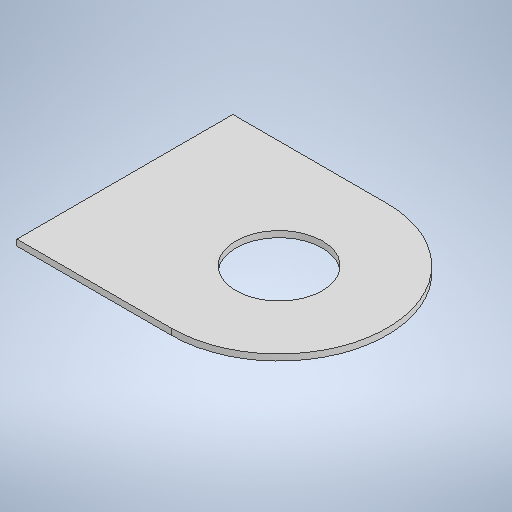
# Autodesk Inventor part: AKVA MSC 0512 transverse ring1 4mm 304 8pcs
Saved by Autodesk Inventor 2025 (Build 290162010, 162A)
## iProperties
Created: 2024-07-11
Part Number: AKVA MSC 0512 transverse ring1 4mm 304 8pcs
Material: Stainless Steel
Document SubType Name: Sheet Metal
Designer: admin
Density: 8 g/cm^3
Sheet Metal Rule: AISI304 2mm Die16
Sheet Metal Width: 85,000 mm
Sheet Metal Length: 70,000 mm
Sheet Metal Area: 5950,000 mm^2
Appearance: Default
Flat Pattern Width: 8.5 cm
Flat Pattern Length: 7 cm
Flat Pattern Area: 59.5 cm^2
Author: admin
Autodesk Inventor part; units mm, degrees
ref_plane "YZ Plane" through (0, 0, 0) normal (1, 0, 0) x (0, 1, 0)
ref_plane "XZ Plane" through (0, 0, 0) normal (0, 1, 0) x (-1, 0, 0)
ref_plane "XY Plane" through (0, 0, 0) normal (0, 0, 1) x (1, 0, 0)
sketch "Sketch1" plane through (0, 0, 0) normal (0, 0, 1) x (1, 0, 0)
  line L0 (0, 35) -> (0, -35)
  line L1 (0, -35) -> (50, -35)
  line L2 (50, 35) -> (0, 35)
  circle A0 centre (50, 0) radius 14
  arc A1 (50, -35) -> (50, 35) centre (50, 0) ccw
  point P0 (0, 0)
  point P1 (0, 0)
  dimension "d11" = 70
  dimension "d12" = 50
  dimension "d14" = 28
  measures "d11" distance of L0.start L0.end
  measures "d12" distance of L0.end L1.end
  measures "d14" diameter of A0
extrude "Plate1" add sketch "Sketch1" along normal blind 2
equation "\"d5\" = Thickness"
equation "\"BendReliefWidth\" = Thickness"
equation "\"BendReliefDepth\" = 0.5 * Thickness"
equation "\"CornerReliefSize\" = 4 * Thickness"
equation "\"MinimumRemnant\" = 2 * Thickness"
equation "\"TransitionRadius\" = BendRadius"
equation "\"JacobiRadiusSize\" = BendRadius"
equation "\"GapSize\" = Thickness"
equation "\"Thickness\" = 2"
equation "\"BendRadius\" = 2.75"
body "Solid1"
